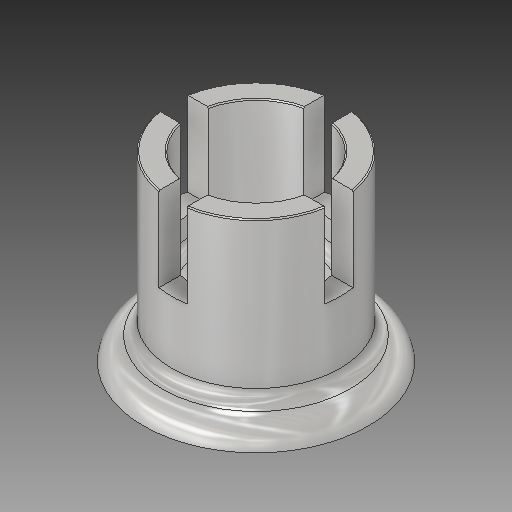
# Autodesk Inventor part: Disco de Apriete
Saved by Autodesk Inventor 2020 (Build 240168000, 168)
## iProperties
Created: 2016-05-09
Part Number: Disco de Apriete
Material: Aluminum 6061-AHC
Document SubType Name: Modeling
Designer: Jorge
Mass: 11.0706 g
Surface Area: 27.4547 cm^2
Volume: 4.10022 cm^3
Density: 2.7 g/cm^3
Appearance: Aluminum - Dark
Author: Jorge
Autodesk Inventor part; units mm, degrees
ref_plane "YZ Plane" through (0, 0, 0) normal (1, 0, 0) x (0, 1, 0)
ref_plane "XZ Plane" through (0, 0, 0) normal (0, 1, 0) x (-1, 0, 0)
ref_plane "XY Plane" through (0, 0, 0) normal (0, 0, 1) x (1, 0, 0)
sketch "Sketch1" plane through (0, 0, 0) normal (0, 0, 1) x (1, 0, 0)
  line L0 (-7.1438, 20.6375) -> (-9.525, 20.6375)
  line L1 (-9.525, 20.6375) -> (-9.525, 4.0656)
  line L2 (-12.7, 0) -> (0, 0)
  line L3 (0, -4.6495) -> (0, 24.852) projected
  line L4 (-7.1438, 20.6375) -> (-7.1437, 8.8537)
  line L5 (-6.3504, 7.4791) -> (0, 3.81)
  line L6 (0, 3.81) -> (0, 0)
  arc A0 (-10.5933, 2.5654) -> (-9.525, 4.0656) centre (-11.1125, 4.0656) ccw
  arc A1 (-10.5933, 2.5654) -> (-12.7, 0) centre (-9.5549, -0.435) ccw
  arc A2 (-7.1437, 8.8537) -> (-6.3504, 7.4791) centre (-5.5563, 8.8537) ccw
  point P0 (-9.525, 3.175)
  point P1 (-7.1437, 7.9375)
  dimension "d0" = 20.6375
  dimension "d1" = 19.05
  dimension "d2" = 14.2875
  dimension "d3" = 12.7
  dimension "d4" = 3.175
  dimension "d5" = 25.4
  dimension "d6" = 1.5875
  dimension "d7" = 3.175
  dimension "d8" = 3.81
  dimension "d10" = 1.5875
  constraints: 12 end point, 6 point on circle, 4 point on line, 4 tangent, 3 centre point, 1 collinear, 1 horizontal, 1 parallel, 1 perpendicular, 1 vertical
  measures "d0" distance from line of L2.end L0
  measures "d1" diameter of L1 L3
  measures "d2" diameter of L4 L3
  measures "d3" distance from line of point (-7.144, 7.938) L0
  measures "d4" distance from line of L2 point (-9.525, 3.175)
  measures "d5" diameter of L2.start L3
  measures "d6" radius of A0
  measures "d7" radius of A1
  measures "d8" distance of L2.end L5.end
  measures "d10" radius of A2
revolve "Revolution1" add sketch "Sketch1" angle 360 about axis through (0, -10, 0) along (0, 1, 0)
chamfer "Chamfer1" distance 0.127 angle 45 2 edges at (9.525, 20.6375, 0) (7.1438, 20.6375, 0)
sketch "Sketch2" plane through (0, 20.6375, 0) normal (0, 1, 0) x (1, 0, 0)
  line L0 (1.5875, 9.6188) -> (1.5875, 6.8545)
  line L1 (1.5875, 6.8545) -> (-1.5875, 6.8545) construction
  line L2 (-1.5875, 6.8545) -> (-1.5875, 9.6188)
  line L3 (0, 17.78) -> (0, -17.78) construction
  arc A0 (1.5875, 9.4869) -> (-1.5875, 9.4869) centre (0, 0) ccw
  arc A1 (1.5875, 6.9651) -> (-1.5875, 6.9651) centre (0, 0) ccw
  dimension "d14" = 3.175
  dimension "d15" = 1.5875
  constraints: 6 end point, 4 point on circle, 4 point on line, 2 centre point, 2 coincident, 1 parallel
  measures "d14" distance between parallel lines of L0 L2
  measures "d15" distance between parallel lines of L3 L2
extrude "Extrusion1" cut sketch "Sketch2" against normal blind 9.525
pattern_circular "Circular Pattern1" count 4 over 360 about axis through (0, -10, 0) along (0, 1, 0) of "Extrusion1"
equation "\"d15\" = 0.5 * d14"
body "Solid1"
